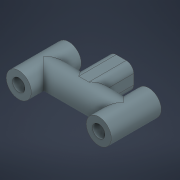
# Autodesk Inventor part: spojka_pol_stredne_koleso
Saved by Autodesk Inventor 2022 (Build 260153000, 153)
## iProperties
Created: 2021-12-17
Part Number: spojka_pol_stredne_koleso
Material: Generic
Document SubType Name: Modeling
Designer: MatusBarany
Density: 1 g/cm^3
Appearance: Default
Author: MatusBarany
Autodesk Inventor part; units mm, degrees
ref_plane "XZ Plane" through (0, 0, 0) normal (0, 1, 0) x (-1, 0, 0)
ref_plane "XY Plane" through (0, 0, 0) normal (0, 0, 1) x (1, 0, 0)
sketch "Sketch1" plane through (0, 0, 0) normal (0, 0, 1) x (1, 0, 0)
  circle A0 centre (0, 0) radius 2.5
  circle A1 centre (0, 0) radius 5
  dimension "d0" = 10
  dimension "d1" = 5
  constraints: 2 centre point, 2 coincident
  measures "d0" diameter of A1
  measures "d1" diameter of A0
extrude "Extrusion1" add sketch "Sketch1" along normal blind 20
ref_plane "Work Plane2" through (-5, 0, 0) normal (1, 0, 0) x (0, 1, 0)
ref_plane "Work Plane1" through (0, 0, 0) normal (1, 0, 0) x (0, 1, 0)
sketch "Sketch2" plane through (-5, 0, 0) normal (1, 0, 0) x (0, 1, 0)
  line L0 (-2.5, 0) -> (2.5, 0) projected
  line L1 (-2.5, 20) -> (2.5, 20) projected
  line L2 (0, 0) -> (0, 20) construction
  circle A0 centre (0, 10) radius 5
  dimension "d6" = 10
  constraints: 2 end point, 2 midpoint, 1 centre point
  measures "d6" diameter of A0
extrude "Extrusion2" cut sketch "Sketch2" along normal blind 5
sketch "Sketch3" plane through (0, 0, 10) normal (-1, 0, 0) x (0, -1, 0)
  circle A0 centre (0, 0) radius 5
  arc A1 (-2.5, 4.3301) -> (-5, 0) centre (0, 0) ccw projected
  point P0 (0, -10)
  point P1 (5, 0)
  point P2 (-3, -4)
  point P3 (3, -4)
  point P4 (2.5, -4.3301)
  point P5 (2.5, 4.3301)
  dimension "d9" = 10
  constraints: 1 centre point, 1 concentric
  measures "d9" diameter of A0
extrude "Extrusion3" add sketch "Sketch3" along normal blind 16
ref_plane "Work Plane4" through (-16, 0, 10) normal (-1, 0, 0) x (0, 0, 1)
sketch "Sketch7" plane through (0, 0, 10) normal (1, 0, 0) x (0, 0, -1)
  line L0 (-4.3301, 2.5) -> (4.3301, 2.5) projected
  arc A0 (-4.3301, 2.5) -> (-4.3301, -2.5) centre (0, 0) ccw projected
  line L1 (4.3301, -2.5) -> (-4.3301, -2.5) projected
  arc A1 (4.3301, -2.5) -> (4.3301, 2.5) centre (0, 0) ccw projected
  point P0 (10, 0)
extrude "Extrusion6" add sketch "Sketch7" along normal blind 4
mirror "Mirror2" about plane through (-16, 0, 10) normal (-1, 0, 0)
ref_plane "Work Plane5" through (0, 0, 5) normal (0, 0, -1) x (-1, 0, 0)
sketch "Sketch8" plane through (0, 0, 5) normal (0, 0, -1) x (-1, 0, 0)
  arc A0 (32, 5) -> (32, -5) centre (32, 0) ccw projected
  arc A1 (32, 5) -> (32, -5) centre (32, 0) ccw projected
  arc A2 (0, -5) -> (0, 5) centre (0, 0) ccw projected
  arc A3 (0, -5) -> (0, 5) centre (0, 0) ccw projected
  line L0 (0, 5) -> (32, 5) projected
  line L1 (11, 5) -> (21, 5)
  line L2 (21, 5) -> (21, -5)
  line L3 (21, -5) -> (11, -5)
  line L4 (11, -5) -> (11, 5)
  line L5 (0, -5) -> (32, -5) projected
  point P0 (0, 0)
  dimension "d33" = 10
  dimension "d34" = 10
  dimension "d35" = 22
  dimension "d36" = 6
  constraints: 8 end point, 2 parallel, 2 point on line, 1 horizontal, 1 perpendicular
  measures "d33" distance between parallel lines of L2 L4
  measures "d34" distance of L1.end L2.end
  measures "d36" distance edge to line of A2 L4
extrude "Extrusion7" add sketch "Sketch8" along normal blind 10 and the other way blind 5 contours L2 L3 L4 L0
fillet "Fillet1" radius 3 4 edges at (-21, 5, 2.5) (-11, 5, 2.5) (-11, -5, 2.5) (-21, -5, 2.5)
sketch "Sketch9" plane through (0, 0, -5) normal (0, 0, -1) x (-1, 0, 0)
  circle A0 centre (16, 0) radius 2.5
  line L0 (21, -2) -> (21, 2) projected
  line L1 (11, 2) -> (11, -2) projected
  line L2 (18, 5) -> (14, 5) projected
  line L3 (14, -5) -> (18, -5) projected
  point P0 (0, 0)
  dimension "d42" = 5
  dimension "d43" = 10
  dimension "d44" = 10
  dimension "d45" = 5
  dimension "d46" = 5
  constraints: 1 centre point
  measures "d42" distance from line of A0.centre L0
  measures "d43" distance between parallel lines of L0 L1
  measures "d44" distance between parallel lines of L2 L3
  measures "d45" distance from line of L2 A0.centre
  measures "d46" diameter of A0
extrude "Extrusion8" cut sketch "Sketch9" against normal blind 5
equation "\"d36\" = -0.5 * d33 + 0.5 * d35"
equation "\"d42\" = 0.5 * d43"
equation "\"d45\" = 0.5 * d44"
equation "\"d5\" = -d1"
body "Solid1"
